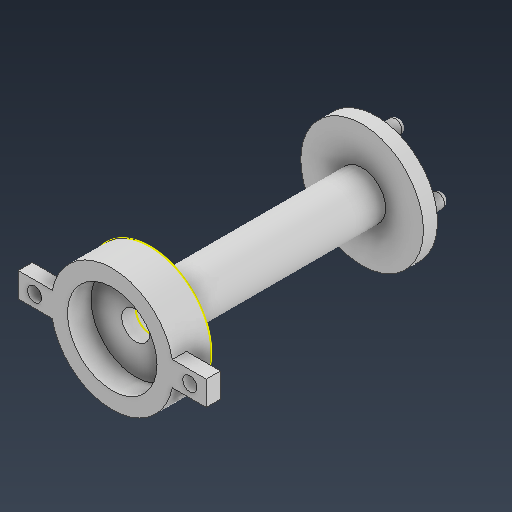
# Autodesk Inventor part: вт1
Saved by Autodesk Inventor 2025 (Build 290162000, 162)
## iProperties
Created: 2025-03-14
Part Number: вт1
Material: Типовые
Document SubType Name: Modeling
Designer: GameHD
Density: 1 g/cm^3
Appearance: По умолчанию
Author: GameHD
Autodesk Inventor part; units mm, degrees
ref_plane "YZ Plane" through (0, 0, 0) normal (1, 0, 0) x (0, 1, 0)
ref_plane "XZ Plane" through (0, 0, 0) normal (0, 1, 0) x (-1, 0, 0)
ref_plane "XY Plane" through (0, 0, 0) normal (0, 0, 1) x (1, 0, 0)
sketch "Эскиз1" plane through (0, 0, 0) normal (0, 0, 1) x (1, 0, 0)
  circle A0 centre (0, 0) radius 3
  circle A1 centre (0, 0) radius 5
  dimension "d0" = 6
  dimension "d1" = 10
  constraints: 2 centre point, 2 coincident
  measures "d0" diameter of A0
  measures "d1" diameter of A1
extrude "Выдавливание1" add sketch "Эскиз1" along normal blind 45
sketch "Эскиз2" plane through (0, 0, 0) normal (0, 0, -1) x (-1, 0, 0)
  circle A0 centre (0, 0) radius 13
  circle A1 centre (0, 0) radius 5 projected
  circle A2 centre (0, 0) radius 3 projected
  dimension "d4" = 26
  constraints: 1 centre point, 1 coincident
  measures "d4" diameter of A0
extrude "Выдавливание2" add sketch "Эскиз2" along normal blind 3 contours A0 | A1
sketch "Эскиз3" plane through (0, 0, -3) normal (0, 0, -1) x (-1, 0, 0)
  circle A0 centre (0, 9) radius 1.5
  circle A1 centre (-9, 0) radius 1.5
  circle A2 centre (0, -9) radius 1.5
  circle A3 centre (9, 0) radius 1.5
  circle A4 centre (0, 0) radius 5 projected
  dimension "d7" = 3
  dimension "d8" = 3
  dimension "d10" = 3
  dimension "d23" = 3
  dimension "d24" = 9
  dimension "d25" = 9
  dimension "d26" = 9
  dimension "d27" = 9
  constraints: 4 centre point
  measures "d7" diameter of A0
  measures "d8" diameter of A1
  measures "d10" diameter of A2
  measures "d23" diameter of A3
  measures "d24" distance of A3.centre point (0, 0)
  measures "d25" distance of A0.centre point (0, 0)
  measures "d26" distance of A4.centre A2.centre
  measures "d27" distance of A1.centre point (0, 0)
extrude "Выдавливание3" add sketch "Эскиз3" along normal blind 5 contours A0 | A1 | A2 | A3
fillet "Сопряжение1" radius 1 4 edges at (1.5, 9, -8) (10.5, 0, -8) (1.5, -9, -8) (-7.5, 0, -8)
sketch "Эскиз4" plane through (0, 0, 45) normal (0, 0, 1) x (1, 0, 0)
  circle A0 centre (0, 9) radius 1.5 projected
  circle A1 centre (0, 0) radius 13 projected
  circle A2 centre (0, 0) radius 5 projected
  circle A3 centre (0, 0) radius 3 projected
  point P0 (-0.5792, 4.9663)
  point P1 (0.5792, 4.9663)
extrude "Выдавливание4" add sketch "Эскиз4" along normal blind 3 contours A0 | A1 | A2
sketch "Эскиз6" plane through (0, 0, 48) normal (0, 0, 1) x (1, 0, 0)
  circle A0 centre (0, 0) radius 9.5
  circle A1 centre (0, 0) radius 13 projected
  dimension "d19" = 19
  constraints: 1 centre point
  measures "d19" diameter of A0
extrude "Выдавливание6" add sketch "Эскиз6" along normal blind 5
sketch "Эскиз8" plane through (0, 0, 53) normal (0, 0, 1) x (1, 0, 0)
  circle A0 centre (-16.4751, 0) radius 1.5
  circle A1 centre (0, 9) radius 1.5
  arc A2 (1.4487, -9.3889) -> (-1.4487, -9.3889) centre (0, -9) ccw
  line L0 (0, 9) -> (0, -9)
  circle A3 centre (0, 0) radius 13
  circle A4 centre (0, 0) radius 9.5
  line L1 (-13, 2.5984) -> (-11.6906, 2.5984)
  line L2 (-13, -2.5984) -> (-12.3453, -2.5984)
  line L3 (-13, -2.5984) -> (-13, 2.5984)
  line L4 (-19.9502, -2.5984) -> (-13, -2.5984)
  line L5 (-19.9502, 2.5984) -> (-19.9502, -2.5984)
  line L6 (-19.9502, -2.5984) -> (-13, 2.5984) construction
  line L7 (-13, -2.5984) -> (-19.9502, 2.5984) construction
  line L8 (-13, 2.5984) -> (-19.9502, 2.5984)
  circle A5 centre (16.4751, 0) radius 1.5
  line L9 (13, 2.5984) -> (11.6906, 2.5984)
  line L10 (13, -2.5984) -> (12.3453, -2.5984)
  line L11 (13, -2.5984) -> (13, 2.5984)
  circle A6 centre (16.4751, 0) radius 1.5
  line L12 (19.9502, -2.5984) -> (13, -2.5984)
  line L13 (13, 2.5984) -> (19.9502, 2.5984)
  line L14 (19.9502, -2.5984) -> (13, 2.5984) construction
  line L15 (13, -2.5984) -> (19.9502, 2.5984) construction
  line L16 (19.9502, 2.5984) -> (19.9502, -2.5984)
  point P0 (12.7377, 2.5984)
  point P1 (12.7377, -2.5984)
  point P2 (-12.7377, -2.5984)
  point P3 (-12.7377, 2.5984)
  dimension "d30" = 3
  constraints: 34 end point, 8 symmetric about line, 7 centre point, 2 horizontal, 2 midpoint, 2 parallel, 2 point on circle, 1 perpendicular, 1 vertical, 2 other
  measures "d30" diameter of A0
extrude "Выдавливание7" add sketch "Эскиз8" against normal blind 3 contours L11 L10 A3 | L11 L13 L16 L12 | A3 L9 L11 | A3 L3 L1 | L2 L3 A3 | L3 L4 L5 L8
